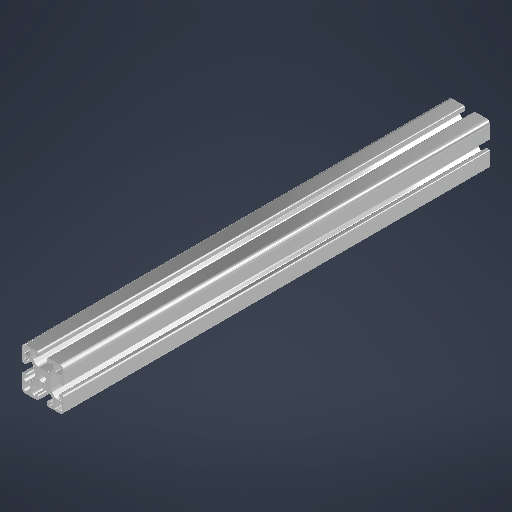
# Autodesk Inventor part: profileAluAvant3
Saved by Autodesk Inventor 2026.2 (Build 302298010, 298A)
## iProperties
Part Number: profileAluAvant3
Material: Générique
Document SubType Name: Modélisation
Designer: quent
Appearance: Par défaut
Author: quent
Autodesk Inventor part; units mm, degrees
ref_plane "Plan YZ" through (0, 0, 0) normal (1, 0, 0) x (0, 1, 0)
ref_plane "Plan XZ" through (0, 0, 0) normal (0, 1, 0) x (-1, 0, 0)
ref_plane "Plan XY" through (0, 0, 0) normal (0, 0, 1) x (1, 0, 0)
sketch "Esquisse1" plane through (0, 0, 0) normal (0, 0, 1) x (1, 0, 0)
  arc A0 (-13.1877, 8.4826) -> (-12.0627, 7.3576) centre (-12.0627, 8.4826) ccw
  line L0 (-10.5627, 7.3576) -> (-12.0627, 7.3576)
  arc A1 (-10.5627, 7.3576) -> (-9.8127, 8.1076) centre (-10.5627, 8.1076) ccw
  line L1 (-9.8127, 9.2326) -> (-9.8127, 8.1076)
  arc A2 (-9.8127, 9.2326) -> (-10.1877, 9.6076) centre (-10.1877, 9.2326) ccw
  line L2 (-11.3127, 9.6076) -> (-10.1877, 9.6076)
  arc A3 (-11.6877, 9.9826) -> (-11.3127, 9.6076) centre (-11.3127, 9.9826) ccw
  arc A4 (-9.8127, 11.8576) -> (-11.6877, 9.9826) centre (-9.8127, 9.9826) ccw
  line L3 (-8.832, 11.8576) -> (-9.8127, 11.8576)
  arc A5 (-6.1804, 10.7593) -> (-8.832, 11.8576) centre (-8.832, 8.1076) ccw
  line L4 (-5.0986, 9.6775) -> (-6.1804, 10.7593)
  arc A6 (-4.0002, 7.0258) -> (-5.0986, 9.6775) centre (-7.7502, 7.0258) ccw
  line L5 (-4.0002, 1.6894) -> (-4.0002, 7.0258)
  arc A7 (-5.0986, -0.9622) -> (-4.0002, 1.6894) centre (-7.7502, 1.6894) ccw
  line L6 (-6.1804, -2.044) -> (-5.0986, -0.9622)
  arc A8 (-8.832, -3.1424) -> (-6.1804, -2.044) centre (-8.832, 0.6076) ccw
  line L7 (-9.8127, -3.1424) -> (-8.832, -3.1424)
  arc A9 (-11.6877, -1.2674) -> (-9.8127, -3.1424) centre (-9.8127, -1.2674) ccw
  arc A10 (-11.3127, -0.8924) -> (-11.6877, -1.2674) centre (-11.3127, -1.2674) ccw
  line L8 (-10.1877, -0.8924) -> (-11.3127, -0.8924)
  arc A11 (-10.1877, -0.8924) -> (-9.8127, -0.5174) centre (-10.1877, -0.5174) ccw
  line L9 (-9.8127, 0.6076) -> (-9.8127, -0.5174)
  arc A12 (-9.8127, 0.6076) -> (-10.5627, 1.3576) centre (-10.5627, 0.6076) ccw
  line L10 (-12.0627, 1.3576) -> (-10.5627, 1.3576)
  arc A13 (-12.0627, 1.3576) -> (-13.1877, 0.2326) centre (-12.0627, 0.2326) ccw
  line L11 (-13.1877, -7.6424) -> (-13.1877, 0.2326)
  arc A14 (-13.1877, -7.6424) -> (-10.1877, -10.6424) centre (-10.1877, -7.6424) ccw
  line L12 (-2.3127, -10.6424) -> (-10.1877, -10.6424)
  arc A15 (-2.3127, -10.6424) -> (-1.1877, -9.5174) centre (-2.3127, -9.5174) ccw
  line L13 (-1.1877, -8.0174) -> (-1.1877, -9.5174)
  arc A16 (-1.1877, -8.0174) -> (-1.9377, -7.2674) centre (-1.9377, -8.0174) ccw
  line L14 (-3.0627, -7.2674) -> (-1.9377, -7.2674)
  arc A17 (-3.0627, -7.2674) -> (-3.4377, -7.6424) centre (-3.0627, -7.6424) ccw
  line L15 (-3.4377, -8.7674) -> (-3.4377, -7.6424)
  arc A18 (-3.8127, -9.1424) -> (-3.4377, -8.7674) centre (-3.8127, -8.7674) ccw
  arc A19 (-5.6877, -7.2674) -> (-3.8127, -9.1424) centre (-3.8127, -7.2674) ccw
  line L16 (-5.6877, -6.2867) -> (-5.6877, -7.2674)
  arc A20 (-4.5894, -3.635) -> (-5.6877, -6.2867) centre (-1.9377, -6.2867) ccw
  line L17 (-3.5076, -2.5532) -> (-4.5894, -3.635)
  arc A21 (-0.8559, -1.4549) -> (-3.5076, -2.5532) centre (-0.8559, -5.2049) ccw
  line L18 (4.4805, -1.4549) -> (-0.8559, -1.4549)
  arc A22 (7.1321, -2.5532) -> (4.4805, -1.4549) centre (4.4805, -5.2049) ccw
  line L19 (8.2139, -3.635) -> (7.1321, -2.5532)
  arc A23 (9.3123, -6.2867) -> (8.2139, -3.635) centre (5.5623, -6.2867) ccw
  line L20 (9.3123, -7.2674) -> (9.3123, -6.2867)
  arc A24 (7.4373, -9.1424) -> (9.3123, -7.2674) centre (7.4373, -7.2674) ccw
  arc A25 (7.0623, -8.7674) -> (7.4373, -9.1424) centre (7.4373, -8.7674) ccw
  line L21 (7.0623, -7.6424) -> (7.0623, -8.7674)
  arc A26 (7.0623, -7.6424) -> (6.6873, -7.2674) centre (6.6873, -7.6424) ccw
  line L22 (5.5623, -7.2674) -> (6.6873, -7.2674)
  arc A27 (5.5623, -7.2674) -> (4.8123, -8.0174) centre (5.5623, -8.0174) ccw
  line L23 (4.8123, -9.5174) -> (4.8123, -8.0174)
  arc A28 (4.8123, -9.5174) -> (5.9373, -10.6424) centre (5.9373, -9.5174) ccw
  line L24 (13.8123, -10.6424) -> (5.9373, -10.6424)
  arc A29 (13.8123, -10.6424) -> (16.8123, -7.6424) centre (13.8123, -7.6424) ccw
  line L25 (16.8123, 0.2326) -> (16.8123, -7.6424)
  arc A30 (16.8123, 0.2326) -> (15.6873, 1.3576) centre (15.6873, 0.2326) ccw
  line L26 (14.1873, 1.3576) -> (15.6873, 1.3576)
  arc A31 (14.1873, 1.3576) -> (13.4373, 0.6076) centre (14.1873, 0.6076) ccw
  line L27 (13.4373, -0.5174) -> (13.4373, 0.6076)
  arc A32 (13.4373, -0.5174) -> (13.8123, -0.8924) centre (13.8123, -0.5174) ccw
  line L28 (14.9373, -0.8924) -> (13.8123, -0.8924)
  arc A33 (15.3123, -1.2674) -> (14.9373, -0.8924) centre (14.9373, -1.2674) ccw
  arc A34 (13.4373, -3.1424) -> (15.3123, -1.2674) centre (13.4373, -1.2674) ccw
  line L29 (12.4566, -3.1424) -> (13.4373, -3.1424)
  arc A35 (9.8049, -2.044) -> (12.4566, -3.1424) centre (12.4566, 0.6076) ccw
  line L30 (8.7231, -0.9622) -> (9.8049, -2.044)
  arc A36 (7.6248, 1.6894) -> (8.7231, -0.9622) centre (11.3748, 1.6894) ccw
  line L31 (7.6248, 7.0258) -> (7.6248, 1.6894)
  arc A37 (8.7231, 9.6775) -> (7.6248, 7.0258) centre (11.3748, 7.0258) ccw
  line L32 (9.8049, 10.7593) -> (8.7231, 9.6775)
  arc A38 (12.4566, 11.8576) -> (9.8049, 10.7593) centre (12.4566, 8.1076) ccw
  line L33 (13.4373, 11.8576) -> (12.4566, 11.8576)
  arc A39 (15.3123, 9.9826) -> (13.4373, 11.8576) centre (13.4373, 9.9826) ccw
  arc A40 (14.9373, 9.6076) -> (15.3123, 9.9826) centre (14.9373, 9.9826) ccw
  line L34 (13.8123, 9.6076) -> (14.9373, 9.6076)
  arc A41 (13.8123, 9.6076) -> (13.4373, 9.2326) centre (13.8123, 9.2326) ccw
  line L35 (13.4373, 8.1076) -> (13.4373, 9.2326)
  arc A42 (13.4373, 8.1076) -> (14.1873, 7.3576) centre (14.1873, 8.1076) ccw
  line L36 (15.6873, 7.3576) -> (14.1873, 7.3576)
  arc A43 (15.6873, 7.3576) -> (16.8123, 8.4826) centre (15.6873, 8.4826) ccw
  line L37 (16.8123, 16.3576) -> (16.8123, 8.4826)
  arc A44 (16.8123, 16.3576) -> (13.8123, 19.3576) centre (13.8123, 16.3576) ccw
  line L38 (5.9373, 19.3576) -> (13.8123, 19.3576)
  arc A45 (5.9373, 19.3576) -> (4.8123, 18.2326) centre (5.9373, 18.2326) ccw
  line L39 (4.8123, 16.7326) -> (4.8123, 18.2326)
  arc A46 (4.8123, 16.7326) -> (5.5623, 15.9826) centre (5.5623, 16.7326) ccw
  line L40 (6.6873, 15.9826) -> (5.5623, 15.9826)
  arc A47 (6.6873, 15.9826) -> (7.0623, 16.3576) centre (6.6873, 16.3576) ccw
  line L41 (7.0623, 17.4826) -> (7.0623, 16.3576)
  arc A48 (7.4373, 17.8576) -> (7.0623, 17.4826) centre (7.4373, 17.4826) ccw
  arc A49 (9.3123, 15.9826) -> (7.4373, 17.8576) centre (7.4373, 15.9826) ccw
  line L42 (9.3123, 15.0019) -> (9.3123, 15.9826)
  arc A50 (8.2139, 12.3503) -> (9.3123, 15.0019) centre (5.5623, 15.0019) ccw
  line L43 (7.1321, 11.2685) -> (8.2139, 12.3503)
  arc A51 (4.4805, 10.1701) -> (7.1321, 11.2685) centre (4.4805, 13.9201) ccw
  line L44 (-0.8559, 10.1701) -> (4.4805, 10.1701)
  arc A52 (-3.5076, 11.2685) -> (-0.8559, 10.1701) centre (-0.8559, 13.9201) ccw
  line L45 (-4.5894, 12.3503) -> (-3.5076, 11.2685)
  arc A53 (-5.6877, 15.0019) -> (-4.5894, 12.3503) centre (-1.9377, 15.0019) ccw
  line L46 (-5.6877, 15.9826) -> (-5.6877, 15.0019)
  arc A54 (-3.8127, 17.8576) -> (-5.6877, 15.9826) centre (-3.8127, 15.9826) ccw
  arc A55 (-3.4377, 17.4826) -> (-3.8127, 17.8576) centre (-3.8127, 17.4826) ccw
  line L47 (-3.4377, 16.3576) -> (-3.4377, 17.4826)
  arc A56 (-3.4377, 16.3576) -> (-3.0627, 15.9826) centre (-3.0627, 16.3576) ccw
  line L48 (-1.9377, 15.9826) -> (-3.0627, 15.9826)
  arc A57 (-1.9377, 15.9826) -> (-1.1877, 16.7326) centre (-1.9377, 16.7326) ccw
  line L49 (-1.1877, 18.2326) -> (-1.1877, 16.7326)
  arc A58 (-1.1877, 18.2326) -> (-2.3127, 19.3576) centre (-2.3127, 18.2326) ccw
  line L50 (-10.1877, 19.3576) -> (-2.3127, 19.3576)
  arc A59 (-10.1877, 19.3576) -> (-13.1877, 16.3576) centre (-10.1877, 16.3576) ccw
  line L51 (-13.1877, 8.4826) -> (-13.1877, 16.3576)
  line L52 (10.6623, -8.9174) -> (10.6623, -4.8674)
  arc A60 (11.0373, -4.4924) -> (10.6623, -4.8674) centre (11.0373, -4.8674) ccw
  line L53 (11.0373, -4.4924) -> (15.0873, -4.4924)
  arc A61 (15.4623, -4.8674) -> (15.0873, -4.4924) centre (15.0873, -4.8674) ccw
  line L54 (15.4623, -4.8674) -> (15.4623, -7.6424)
  arc A62 (13.8123, -9.2924) -> (15.4623, -7.6424) centre (13.8123, -7.6424) ccw
  line L55 (13.8123, -9.2924) -> (11.0373, -9.2924)
  arc A63 (10.6623, -8.9174) -> (11.0373, -9.2924) centre (11.0373, -8.9174) ccw
  line L56 (-11.4627, -4.4924) -> (-7.4127, -4.4924)
  arc A64 (-7.0377, -4.8674) -> (-7.4127, -4.4924) centre (-7.4127, -4.8674) ccw
  line L57 (-7.0377, -4.8674) -> (-7.0377, -8.9174)
  arc A65 (-7.4127, -9.2924) -> (-7.0377, -8.9174) centre (-7.4127, -8.9174) ccw
  line L58 (-7.4127, -9.2924) -> (-10.1877, -9.2924)
  arc A66 (-11.8377, -7.6424) -> (-10.1877, -9.2924) centre (-10.1877, -7.6424) ccw
  line L59 (-11.8377, -7.6424) -> (-11.8377, -4.8674)
  arc A67 (-11.4627, -4.4924) -> (-11.8377, -4.8674) centre (-11.4627, -4.8674) ccw
  line L60 (-7.0377, 17.6326) -> (-7.0377, 13.5826)
  arc A68 (-7.4127, 13.2076) -> (-7.0377, 13.5826) centre (-7.4127, 13.5826) ccw
  line L61 (-7.4127, 13.2076) -> (-11.4627, 13.2076)
  arc A69 (-11.8377, 13.5826) -> (-11.4627, 13.2076) centre (-11.4627, 13.5826) ccw
  line L62 (-11.8377, 13.5826) -> (-11.8377, 16.3576)
  arc A70 (-10.1877, 18.0076) -> (-11.8377, 16.3576) centre (-10.1877, 16.3576) ccw
  line L63 (-10.1877, 18.0076) -> (-7.4127, 18.0076)
  arc A71 (-7.0377, 17.6326) -> (-7.4127, 18.0076) centre (-7.4127, 17.6326) ccw
  line L64 (15.0873, 13.2076) -> (11.0373, 13.2076)
  arc A72 (10.6623, 13.5826) -> (11.0373, 13.2076) centre (11.0373, 13.5826) ccw
  line L65 (10.6623, 13.5826) -> (10.6623, 17.6326)
  arc A73 (11.0373, 18.0076) -> (10.6623, 17.6326) centre (11.0373, 17.6326) ccw
  line L66 (11.0373, 18.0076) -> (13.8123, 18.0076)
  arc A74 (15.4623, 16.3576) -> (13.8123, 18.0076) centre (13.8123, 16.3576) ccw
  line L67 (15.4623, 16.3576) -> (15.4623, 13.5826)
  arc A75 (15.0873, 13.2076) -> (15.4623, 13.5826) centre (15.0873, 13.5826) ccw
  circle A76 centre (1.8123, 4.3576) radius 2.55
  point P0 (0, 0)
  point P1 (-13.078, -1.9686)
  point P2 (-1.7532, 3.3389)
  point P3 (-1.1377, 8.1076)
  constraints: 152 point on circle, 136 end point, 77 centre point
extrude "Extrusion1" add sketch "Esquisse1" along normal blind 301.624
